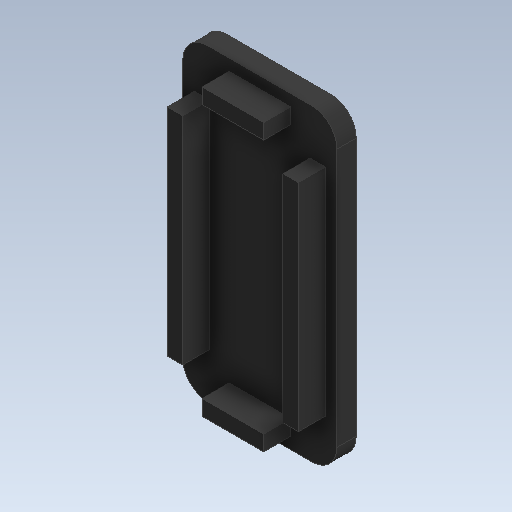
# Autodesk Inventor part: SP18V1 Tapacanto Superior
Saved by Autodesk Inventor 2021.2 (Build 252289000, 289)
## iProperties
Created: 2026-06-08
Part Number: SP18V1 Tapacanto Superior
Material: Generic
Document SubType Name: Modeling
Designer: NELSON
Density: 1 g/cm^3
Appearance: Default
Author: NELSON
Autodesk Inventor part; units mm, degrees
ref_plane "YZ Plane" through (0, 0, 0) normal (1, 0, 0) x (0, 1, 0)
ref_plane "XZ Plane" through (0, 0, 0) normal (0, 1, 0) x (-1, 0, 0)
ref_plane "XY Plane" through (0, 0, 0) normal (0, 0, 1) x (1, 0, 0)
sketch "Boceto1" plane through (0, 0, 0) normal (0, 0, 1) x (1, 0, 0)
  line L0 (20, -40) -> (-20, -40)
  line L1 (-20, -40) -> (-20, 40)
  line L2 (-20, 40) -> (20, 40)
  line L3 (20, 40) -> (20, -40)
  line L4 (20, -40) -> (-20, 40) construction
  line L5 (-20, -40) -> (20, 40) construction
  point P0 (0, 0)
  dimension "d0" = 40
  dimension "d22" = 80
  constraints: 12 end point, 2 midpoint, 2 parallel, 1 horizontal, 1 perpendicular
  measures "d0" distance of L1.end L2.end
  measures "d22" distance of L0.end L1.end
extrude "Extrusión1" add sketch "Boceto1" along normal blind 5
sketch "Boceto2" plane through (0, 0, 5) normal (0, 0, 1) x (1, 0, 0)
  line L0 (17.5, -37.5) -> (-17.5, -37.5)
  line L1 (-17.5, -37.5) -> (-17.5, 37.5)
  line L2 (-17.5, 37.5) -> (17.5, 37.5)
  line L3 (17.5, 37.5) -> (17.5, -37.5)
  line L4 (17.5, -37.5) -> (-17.5, 37.5) construction
  line L5 (-17.5, -37.5) -> (17.5, 37.5) construction
  line L6 (17, 37) -> (-17, 37)
  line L7 (-17, 37) -> (-17, -37)
  line L8 (-17, -37) -> (17, -37)
  line L9 (17, -37) -> (17, 37)
  line L10 (-13, 33) -> (13, 33)
  line L11 (13, 33) -> (13, -33)
  line L12 (13, -33) -> (-13, -33)
  line L13 (-13, -33) -> (-13, 33)
  line L14 (8, 33) -> (8, 37)
  line L15 (-8, 33) -> (-8, 37)
  line L16 (13, 28) -> (17, 28)
  line L17 (13, -28) -> (17, -28)
  line L18 (-13, -28) -> (-17, -28)
  line L19 (-8, -33) -> (-8, -37)
  line L20 (8, -33) -> (8, -37)
  line L21 (-17, 28) -> (-13, 28)
  point P0 (0, 0)
  dimension "d5" = 35
  dimension "d6" = 75
  dimension "d7" = 0.5
  dimension "d8" = 4
  dimension "d9" = 5
  dimension "d10" = 5
  dimension "d11" = 5
  dimension "d12" = 5
  dimension "d13" = 5
  dimension "d14" = 5
  dimension "d15" = 5
  dimension "d16" = 5
  constraints: 44 end point, 16 point on line, 9 perpendicular, 8 parallel, 2 midpoint, 1 horizontal, 6 other
  measures "d5" distance of L1.end L2.end
  measures "d6" distance of L0.end L1.end
  measures "d7" distance between parallel lines of L2 L6
  measures "d8" distance between parallel lines of L6 L10
  measures "d9" distance between parallel lines of L11 L14
  measures "d10" distance between parallel lines of L15 L13
  measures "d11" distance between parallel lines of L16 L10
  measures "d12" distance between parallel lines of L12 L17
  measures "d13" distance between parallel lines of L11 L20
  measures "d14" distance between parallel lines of L13 L19
  measures "d15" distance between parallel lines of L12 L18
  measures "d16" distance between parallel lines of L10 L21
extrude "Extrusión2" add sketch "Boceto2" along normal blind 7 contours L14 L10 L15 L6 | L9 L17 L11 L16 | L21 L13 L18 L7 | L8 L19 L12 L20
fillet "Empalme3" radius 6.5 4 edges at (20, 40, 2.5) (-20, 40, 2.5) (20, -40, 2.5) (-20, -40, 2.5)
